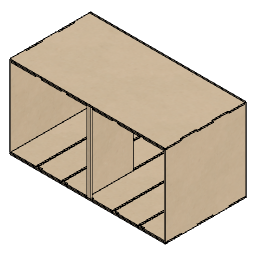
IOIO_Educational_Library (Autodesk Fusion 360 design; units mm, degrees)
Autodesk Fusion 360 part; units mm, degrees
sketch "Bottom_Plate" plane through (0, 0, 0) normal (0, 0, 1) x (1, 0, 0)
  line L0 (195, 100) -> (-195, 100)
  line L1 (-195, 100) -> (-195, -100)
  line L2 (-195, -100) -> (195, -100)
  line L3 (195, -100) -> (195, 100)
  line L4 (195, 100) -> (-195, -100) construction
  line L5 (-195, 100) -> (195, -100) construction
  line L6 (-195, 100) -> (-192, 100)
  line L7 (-192, 100) -> (-192, 60)
  line L8 (-192, 60) -> (-195, 60)
  line L9 (-195, 60) -> (-195, 100)
  line L10 (-192, 60) -> (-192, 20)
  line L11 (-192, 20) -> (-195, 20)
  line L12 (-192, 20) -> (-192, -20)
  line L13 (-192, -20) -> (-195, -20)
  line L14 (-192, -20) -> (-192, -60)
  line L15 (-192, -60) -> (-195, -60)
  line L16 (-192, -60) -> (-192, -100)
  line L17 (-192, -100) -> (-195, -100)
  line L18 (0, 100) -> (0, -100) construction
  line L19 (192, 100) -> (192, 60)
  line L20 (192, 60) -> (195, 60)
  line L21 (192, 60) -> (192, 20)
  line L22 (192, 20) -> (195, 20)
  line L23 (192, 20) -> (192, -20)
  line L24 (192, -20) -> (192, -60)
  line L25 (192, -20) -> (195, -20)
  line L26 (192, -60) -> (195, -60)
  line L27 (192, -60) -> (192, -100)
  dimension "d1" = 390
  dimension "d2" = 200
  dimension "d5" = 3
  dimension "d6" = 40
  dimension "d9" = 160
  dimension "d10" = 0
  constraint horizontal L0
  constraint perpendicular L0 L1
  constraint parallel L0 L2
  constraint parallel L1 L3
  constraint coincident L4 origin
  constraint coincident L5 origin
  constraint horizontal L6
  constraint vertical L7
  constraint horizontal L8
  constraint vertical L9
  constraint midpoint L0 L18.start
  constraint midpoint L2 L18.end
  constraint symmetric L6.end L18 L19.start
  constraint symmetric L7.end L18 L19.end
  constraint symmetric L8.end L18 L20.end
  constraint symmetric L10.end L18 L21.end
  constraint symmetric L11.end L18 L22.end
  constraint symmetric L12.end L18 L23.end
  constraint symmetric L13.end L18 L25.end
  constraint symmetric L14.end L18 L24.end
  constraint symmetric L15.end L18 L26.end
  constraint symmetric L16.end L18 L27.end
  measures "d1" distance of L1.end L2.end
  measures "d2" distance of L0.end L1.end
  measures "d5" distance of L0.end L6.end
  measures "d6" distance of L0.end L8.end
extrude "Extrude2" add sketch "Bottom_Plate" along normal blind 3 contours L0 L2 L7 L10 L12 L14 L16 L19 L21 L23 L24 L27 makes body 1
extrude "Extrude3" add sketch "Bottom_Plate" along normal blind 3 contours L0 L3 L19 L20 | L0 L1 L6 L7 L8 L9 | L3 L22 L23 L25 | L1 L11 L12 L13 | L2 L3 L26 L27 | L1 L2 L15 L16 L17 bodies 1
copy_body "Body->Comp1" bodies 1 removing the originals makes body 2 in component "Library_Body"
copy_body "CopyPasteBodies1" bodies 2 makes body 3 in component "Library_Body"
move_body "Move1" bodies 3 to x (1, 0, 0) y (0, 1, 0) z (0, 0, 1) at (0, 0, 208) in component "Library_Body"
ref_plane "WorkPlane1" through (195, 0, 0) normal (1, 0, 0) x (0, 1, 0) in component "Library_Body"
sketch "Side_Plate" plane through (195, 0, 0) normal (1, 0, 0) x (0, 1, 0) in component "Library_Body"
  line L0 (100, 0) -> (-100, 0)
  line L1 (-100, 0) -> (-100, 207)
  line L2 (-100, 207) -> (100, 207)
  line L3 (100, 207) -> (100, 0)
  line L4 (100, 204) -> (60, 204)
  line L5 (60, 204) -> (60, 207)
  line L6 (60, 207) -> (100, 207)
  line L7 (100, 207) -> (100, 204)
  line L8 (60, 204) -> (20, 204)
  line L9 (20, 204) -> (20, 207)
  line L10 (20, 204) -> (-20, 204)
  line L11 (-20, 204) -> (-20, 207)
  line L12 (-20, 204) -> (-60, 204)
  line L13 (-60, 204) -> (-60, 207)
  line L14 (-60, 204) -> (-100, 204)
  line L15 (-100, 204) -> (-100, 207)
  line L16 (100, 103.5) -> (-100, 103.5) construction
  line L17 (100, 3) -> (60, 3)
  line L18 (60, 3) -> (60, 0)
  line L19 (60, 3) -> (20, 3)
  line L20 (20, 3) -> (20, 0)
  line L21 (20, 3) -> (-20, 3)
  line L22 (-20, 3) -> (-20, 0)
  line L23 (-20, 3) -> (-60, 3)
  line L24 (-60, 3) -> (-60, 0)
  line L25 (-60, 3) -> (-100, 3)
  dimension "d21" = -160
  dimension "d22" = 0
  dimension "d85" = 201
  constraint horizontal L0
  constraint vertical L1
  constraint horizontal L2
  constraint vertical L3
  constraint horizontal L4
  constraint vertical L5
  constraint horizontal L6
  constraint vertical L7
  constraint coincident L2 L5.end
  constraint coincident L3 L4.start
  constraint midpoint L3 L16.start
  constraint midpoint L1 L16.end
  constraint symmetric L4.start L16 L17.start
  constraint symmetric L4.end L16 L17.end
  constraint symmetric L5.end L16 L18.end
  constraint symmetric L8.end L16 L19.end
  constraint symmetric L9.end L16 L20.end
  constraint symmetric L10.end L16 L21.end
  constraint symmetric L11.end L16 L22.end
  constraint symmetric L12.end L16 L23.end
  constraint symmetric L13.end L16 L24.end
  constraint symmetric L14.end L16 L25.end
  measures "d85" distance of L14.end L25.end
extrude "Extrude1" add sketch "Side_Plate" against normal blind 3 separate body contours L1 L3 L4 L8 L10 L12 L14 L17 L19 L21 L23 L25 makes body 4 in component "Library_Body"
extrude "Extrude2'" add sketch "Side_Plate" against normal blind 3 contours L0 L18 L19 L20 | L0 L22 L23 L24 | L2 L5 L8 L9 | L2 L11 L12 L13 bodies 4 in component "Library_Body"
copy_body "CopyPasteBodies2" bodies 4 makes body 5 in component "Library_Body"
move_body "Move2" bodies 5 to x (1, 0, 0) y (0, 1, 0) z (0, 0, 1) at (-387, 0, 0) in component "Library_Body"
sketch "Sketch3" plane through (0, 0, 3) normal (0, 0, 1) x (-1, 0, 0) in component "Library_Body"
  line L0 (-195, -100) -> (195, -100)
  line L1 (195, -100) -> (195, -60)
  line L2 (195, -60) -> (192, -60)
  line L3 (192, -60) -> (192, -20)
  line L4 (192, -20) -> (195, -20)
  line L5 (195, -20) -> (195, 20)
  line L6 (195, 20) -> (192, 20)
  line L7 (192, 20) -> (192, 60)
  line L8 (192, 60) -> (195, 60)
  line L9 (195, 60) -> (195, 100)
  line L10 (195, 100) -> (-195, 100)
  line L11 (-195, 100) -> (-195, 60)
  line L12 (-195, 60) -> (-192, 60)
  line L13 (-192, 60) -> (-192, 20)
  line L14 (-192, 20) -> (-195, 20)
  line L15 (-195, 20) -> (-195, -20)
  line L16 (-195, -20) -> (-192, -20)
  line L17 (-192, -20) -> (-192, -60)
  line L18 (-192, -60) -> (-195, -60)
  line L19 (-195, -60) -> (-195, -100)
  line L20 (192, -60) -> (192, -100) construction
  line L21 (192, -100) -> (130, -100)
  line L22 (130, -100) -> (130, 100)
  line L23 (130, 100) -> (192, 100)
  line L24 (192, 100) -> (192, -100)
  line L25 (-192, -60) -> (-192, -100) construction
  line L26 (-192, -100) -> (-130, -100)
  line L27 (-130, -100) -> (-130, 100)
  line L28 (-130, 100) -> (-192, 100)
  line L29 (-192, 100) -> (-192, -100)
  line L30 (130, -100) -> (126, -100) construction
  line L31 (126, -100) -> (66, -100)
  line L32 (66, -100) -> (66, 100)
  line L33 (66, 100) -> (126, 100)
  line L34 (126, 100) -> (126, -100)
  line L35 (62, -100) -> (2, -100)
  line L36 (2, -100) -> (2, 100)
  line L37 (62, 100) -> (62, -100)
  line L38 (-2, -100) -> (-62, -100)
  line L39 (-62, -100) -> (-62, 100)
  line L40 (-2, 100) -> (-2, -100)
  line L41 (-66, -100) -> (-126, -100)
  line L42 (-126, -100) -> (-126, 100)
  line L43 (-66, 100) -> (-66, -100)
  line L44 (126, 100) -> (116, 100)
  line L45 (116, 100) -> (116, 97)
  line L46 (116, 97) -> (126, 97)
  line L47 (126, 97) -> (126, 100)
  line L48 (52, 97) -> (62, 97)
  line L49 (52, 100) -> (52, 97)
  line L50 (-12, 97) -> (-2, 97)
  line L51 (-12, 100) -> (-12, 97)
  line L52 (-76, 97) -> (-66, 97)
  line L53 (-76, 100) -> (-76, 97)
  line L54 (-140, 97) -> (-130, 97)
  line L55 (-140, 100) -> (-140, 97)
  line L56 (192, -97) -> (130, -97)
  line L57 (126, -97) -> (66, -97)
  line L58 (62, -97) -> (2, -97)
  line L59 (-2, -97) -> (-62, -97)
  line L60 (-66, -97) -> (-126, -97)
  line L61 (-192, -97) -> (-130, -97)
  dimension "d27" = 62
  dimension "d28" = 200
  dimension "d29" = 62
  dimension "d30" = 200
  dimension "d31" = 4
  dimension "d32" = 60
  dimension "d33" = 200
  dimension "d36" = -192
  dimension "d37" = 0
  dimension "d38" = 10
  dimension "d39" = 3
  dimension "d42" = 256
  dimension "d43" = 0
  dimension "d46" = 3
  dimension "d47" = 3
  dimension "d48" = 3
  dimension "d49" = 3
  dimension "d50" = 3
  dimension "d51" = -3
  constraint coincident L2.end L3.start
  constraint coincident L0 L20.end
  constraint perpendicular L0 L20
  constraint horizontal L21
  constraint vertical L22
  constraint horizontal L23
  constraint vertical L24
  constraint coincident L17.end L18.start
  constraint coincident L0 L25.end
  constraint perpendicular L0 L25
  constraint horizontal L26
  constraint vertical L27
  constraint horizontal L28
  constraint vertical L29
  constraint perpendicular L22 L30
  constraint horizontal L31
  constraint vertical L32
  constraint horizontal L33
  constraint vertical L34
  constraint horizontal L44
  constraint vertical L45
  constraint horizontal L46
  constraint vertical L47
  measures "d27" distance of L20.end L21.end
  measures "d28" distance of L20.end L23.end
  measures "d29" distance of L25.end L26.end
  measures "d30" distance of L25.end L28.end
  measures "d31" distance of L21.end L30.end
  measures "d32" distance of L30.end L31.end
  measures "d33" distance of L30.end L33.end
  measures "d38" distance of L33.end L44.end
  measures "d39" distance of L33.end L46.end
extrude "Extrude4" add sketch "Sketch3" along normal blind 3 separate body contours L10 L13 L17 L27 L28 L29 L54 L55 L61 | L10 L42 L43 L52 L53 L60 | L10 L39 L40 L50 L51 L59 | L10 L36 L37 L48 L49 L58 | L10 L32 L33 L34 L45 L46 L57 | L3 L7 L10 L22 L23 L24 L56 makes body 6 at (25.3333, 32.3333, 3) makes body 7 at (-150.6667, 31.3333, 3) makes body 8 at (89.3333, 32.3333, 3) makes body 9 at (-38.6667, 32.3333, 3) makes body 10 at (-102.6667, 32.3333, 3) makes body 11 at (154, 32.3333, 3) in component "Library_Body"
sketch "Back_Plate" plane through (0, 100, 0) normal (0, 1, 0) x (-1, 0, 0) in component "Library_Body"
  line L0 (-195, 0) -> (195, 0)
  line L1 (195, 0) -> (195, 3)
  line L2 (195, 3) -> (-195, 3)
  line L3 (-195, 3) -> (-195, 0)
  line L4 (-195, 207) -> (195, 207)
  line L5 (195, 207) -> (195, 0)
  line L6 (195, 0) -> (-195, 0)
  line L7 (-195, 0) -> (-195, 207)
  line L8 (192, 3) -> (-192, 3)
  line L9 (-192, 3) -> (-192, 204)
  line L10 (-192, 204) -> (192, 204)
  line L11 (192, 204) -> (192, 3)
  line L12 (0, 207) -> (0, 0) construction
  line L13 (195, 103.5) -> (-195, 103.5) construction
  line L14 (192, 204) -> (172, 204)
  line L15 (172, 204) -> (172, 201)
  line L16 (192, 204) -> (192, 184)
  line L17 (192, 184) -> (189, 184)
  line L18 (189, 184) -> (172, 201)
  line L19 (172, 3) -> (172, 6)
  line L20 (189, 23) -> (172, 6)
  line L21 (192, 23) -> (189, 23)
  line L22 (-172, 204) -> (-172, 201)
  line L23 (-189, 184) -> (-172, 201)
  line L24 (-192, 184) -> (-189, 184)
  line L25 (-192, 23) -> (-189, 23)
  line L26 (-189, 23) -> (-172, 6)
  line L27 (-172, 3) -> (-172, 6)
  dimension "d54" = 390
  dimension "d55" = 207
  dimension "d56" = 3
  dimension "d86" = 20
  dimension "d87" = 3
  dimension "d88" = 20
  dimension "d89" = 3
  constraint horizontal L4
  constraint vertical L5
  constraint horizontal L6
  constraint vertical L7
  constraint coincident L0.end L1.start
  constraint midpoint L4 L12.start
  constraint coincident L12.end origin
  constraint midpoint L5 L13.start
  constraint midpoint L7 L13.end
  constraint perpendicular L11 L14
  constraint perpendicular L10 L15
  constraint perpendicular L14 L16
  constraint perpendicular L16 L17
  constraint symmetric L13 L14.end L19.start
  constraint symmetric L13 L15.end L19.end
  constraint symmetric L13 L16.end L21.start
  constraint symmetric L13 L17.end L20.start
  constraint symmetric L12 L14.end L22.start
  constraint symmetric L12 L15.end L22.end
  constraint symmetric L12 L16.end L24.start
  constraint symmetric L12 L17.end L23.start
  constraint symmetric L12 L19.start L27.start
  constraint symmetric L12 L19.end L26.end
  constraint symmetric L12 L20.start L25.end
  constraint symmetric L12 L21.start L25.start
  measures "d54" distance of L4.start L4.end
  measures "d55" distance of L0.start L4.start
  measures "d86" distance of L10.end L14.end
  measures "d87" distance of L14.end L15.end
  measures "d88" distance of L10.end L16.end
  measures "d89" distance of L16.end L17.end
extrude "Extrude5" add sketch "Back_Plate" along normal blind 3 separate body makes body 12 in component "Library_Body"
copy_body "CopyPasteBodies3" bodies 11 7 8 9 10 6 makes body 13 makes body 14 makes body 15 makes body 16 makes body 17 makes body 18 in component "Library_Body"
move_body "Move3" bodies 13 14 15 16 17 18 to x (1, 0, 0) y (0, 1, 0) z (0, 0, 1) at (0, 0, 198) in component "Library_Body"
sketch "Sketch5" plane through (0, 0, 0) normal (0, 0, 1) x (1, 0, 0)
  line L0 (55, -100) -> (-55, -100)
  line L1 (-55, -100) -> (-55, 100)
  line L2 (-55, 100) -> (55, 100)
  line L3 (55, 100) -> (55, -100)
  line L4 (55, -100) -> (-55, 100) construction
  line L5 (-55, -100) -> (55, 100) construction
  dimension "d65" = 110
  dimension "d66" = 200
  constraint horizontal L0
  constraint perpendicular L0 L1
  constraint parallel L0 L2
  constraint parallel L1 L3
  constraint coincident L4 origin
  constraint coincident L5 origin
  measures "d65" distance of L1.end L2.end
  measures "d66" distance of L0.end L1.end
extrude "Extrude7" add sketch "Sketch5" along normal blind 3 separate body makes body 19 in component "Library_Body"
copy_body "Body->Comp1'" bodies 19 removing the originals makes body 20 in component "Module"
sketch "Sketch6" plane through (0, 0, 3) normal (0, 0, 1) x (-1, 0, 0) in component "Library_Body"
  line L0 (-55, -100) -> (55, -100)
  line L1 (55, -100) -> (55, 100)
  line L2 (55, 100) -> (-55, 100)
  line L3 (-55, 100) -> (-55, -100)
  line L4 (47.5, -30) -> (-47.5, -30)
  line L5 (-47.5, -30) -> (-47.5, -95)
  line L6 (-47.5, -95) -> (47.5, -95)
  line L7 (47.5, -95) -> (47.5, -30)
  line L8 (42.5, -90) -> (42.5, -82)
  line L9 (42.5, -90) -> (34.5, -90)
  line L10 (34.5, -90) -> (34.5, -91)
  line L11 (34.5, -91) -> (0, -91)
  line L12 (0, -62.5) -> (45, -62.5) construction
  line L13 (42.5, -82) -> (43.5, -82)
  line L14 (43.5, -82) -> (43.5, -62.5)
  line L15 (0, -100) -> (0, -49) construction
  line L16 (34.5, -90) -> (42.5, -90)
  line L17 (-34.5, -91) -> (0, -91)
  line L18 (-34.5, -90) -> (-34.5, -91)
  line L19 (-34.5, -90) -> (-42.5, -90)
  line L20 (-42.5, -90) -> (-42.5, -82)
  line L21 (-42.5, -82) -> (-43.5, -82)
  line L22 (-43.5, -82) -> (-43.5, -62.5)
  line L23 (34.5, -35) -> (42.5, -35)
  line L24 (-34.5, -35) -> (-34.5, -34)
  line L25 (34.5, -35) -> (34.5, -34)
  line L26 (43.5, -43) -> (43.5, -62.5)
  line L27 (34.5, -34) -> (0, -34)
  line L28 (-42.5, -43) -> (-43.5, -43)
  line L29 (-34.5, -34) -> (0, -34)
  line L30 (-43.5, -43) -> (-43.5, -62.5)
  line L31 (42.5, -43) -> (43.5, -43)
  line L32 (-34.5, -35) -> (-42.5, -35)
  line L33 (-42.5, -35) -> (-42.5, -43)
  line L34 (42.5, -35) -> (34.5, -35)
  line L35 (42.5, -35) -> (42.5, -43)
  line L36 (0, -25) -> (0, -76) construction
  point P0 (0, -62.5)
  dimension "d75" = 8
  dimension "d76" = 8
  dimension "d77" = 1
  dimension "d78" = 1
  constraint perpendicular L8 L9
  constraint perpendicular L10 L11
  constraint coincident P0 L12.start
  constraint coincident L12 L14.end
  constraint perpendicular L12 L14
  constraint midpoint L0 L15.start
  constraint perpendicular L0 L15
  constraint symmetric L8.start L15 L19.end
  constraint symmetric L8.end L15 L20.end
  constraint symmetric L9.end L15 L18.start
  constraint symmetric L10.end L15 L17.start
  constraint symmetric L11.end L15 L17.end
  constraint symmetric L13.end L15 L21.end
  constraint symmetric L14.end L15 L22.end
  constraint symmetric L8.start L12 L23.end
  constraint symmetric L8.end L12 L31.start
  constraint symmetric L9.end L12 L23.start
  constraint symmetric L10.end L12 L25.end
  constraint symmetric L11.end L12 L27.end
  constraint symmetric L12 L13.end L26.start
  constraint symmetric L12 L14.end L26.end
  constraint symmetric L12 L15.start L36.start
  constraint symmetric L12 L15.end L36.end
  constraint symmetric L12 L17.start L24.end
  constraint symmetric L12 L11.end L27.end
  constraint symmetric L12 L18.start L24.start
  constraint symmetric L12 L19.end L32.end
  constraint symmetric L12 L20.end L28.start
  constraint symmetric L12 L21.end L28.end
  constraint symmetric L12 L22.end L30.end
  measures "d75" distance of L8.start L8.end
  measures "d76" distance of L8.start L9.end
  measures "d77" distance of L9.end L10.end
  measures "d78" distance of L8.end L13.end
extrude "Extrude8" add sketch "Sketch6" along normal blind 3 separate body contours L4 L5 L6 L7 makes body 21 in component "Library_Body"
sketch "Sketch8" plane through (-55, 0, 0) normal (-1, 0, 0) x (0, -1, 0) in component "Library_Body"
  line L0 (-100, 0) -> (100, 0)
  line L1 (100, 0) -> (100, 3)
  line L2 (100, 3) -> (-100, 3)
  line L3 (-100, 3) -> (-100, 0)
  line L4 (100, 3) -> (-100, 3)
  line L5 (-100, 3) -> (-100, -7)
  line L6 (-100, -7) -> (100, -7)
  line L7 (100, -7) -> (100, 3)
  dimension "d81" = 200
  dimension "d82" = 10
  constraint horizontal L4
  constraint vertical L5
  constraint horizontal L6
  constraint vertical L7
  constraint coincident L1.end L2.start
  measures "d81" distance of L1.end L2.end
  measures "d82" distance of L1.end L6.end
extrude "Extrude9" add sketch "Sketch8" along normal blind 3 separate body makes body 22 in component "Library_Body"
copy_body "CutPasteBodies1" bodies 21 22 removing the originals makes body 23 makes body 24 in component "Module"
move_body "Move4" bodies 3 to x (1, 0, 0) y (0, 1, 0) z (0, 0, 1) at (0, 0, -4) in component "Library_Body"
extrude "Extrude10" add sketch "Back_Plate" against normal blind 3 separate body contours L2 L8 L9 L25 L26 L27 | L2 L8 L11 L19 L20 L21 | L9 L10 L22 L23 L24 | L10 L11 L14 L15 L16 L17 L18 makes body 25 at (-184.3333, 100, 196.3333) makes body 26 at (184.3333, 100, 10.6667) makes body 27 at (184.3333, 100, 196.3333) makes body 28 at (-184.3333, 100, 10.6667) in component "Library_Body"
component "Library_Body" placed x (1, 0, 0) y (0, 1, 0) z (0, 0, 1) at (0, 0, 0)
component "Module" placed x (1, 0, 0) y (0, 1, 0) z (0, 0, 1) at (0, 0, 0) in component "Library_Body"
equation "d18 = ( 390 / 2 ) * 1 mm"
equation "d55 = 211 mm - 4 mm"
named bodies: "Bottom_Plate", "Bottom_Plate (1)", "Top_Plate", "Right_Plate", "Side_plate", "Left_Plate", "Card_Spacer_Bottom_4", "Card_Spacer_Bottom_1", "Card_Spacer_Bottom_5", "Card_Spacer_Bottom_3", "Card_Spacer_Bottom_2", "Card_Spacer_Bottom_6", "Back_Plate", "Card_Spacer_Top_6", "Card_Spacer_Top_1", "Card_Spacer_Top_5", "Card_Spacer_Top_3", "Card_Spacer_Top_2", "Card_Spacer_Top_4", "Module", "Card_Body", "Breadboard_Slot", "Card_Lip"
